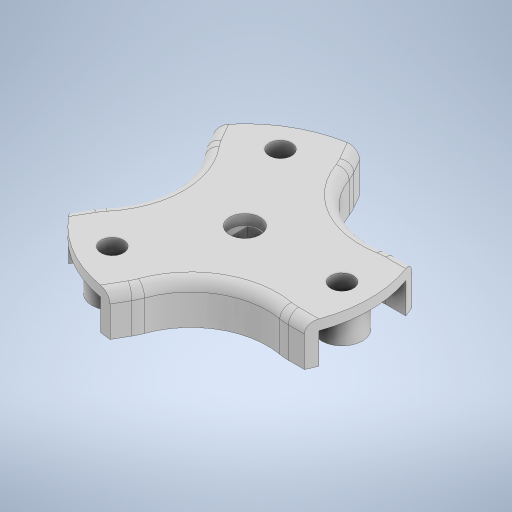
# Autodesk Inventor part: Soporte rodamientos
Saved by Autodesk Inventor 2023 (Build 270158000, 158)
## iProperties
Created: 2023-04-01
Part Number: Soporte rodamientos
Material: Genérico
Document SubType Name: Modeling
Designer: sergi
Density: 1 g/cm^3
Appearance: Valor por defecto
Author: sergi
Autodesk Inventor part; units mm, degrees
ref_plane "YZ Plane" through (0, 0, 0) normal (1, 0, 0) x (0, 1, 0)
ref_plane "XZ Plane" through (0, 0, 0) normal (0, 1, 0) x (-1, 0, 0)
ref_plane "XY Plane" through (0, 0, 0) normal (0, 0, 1) x (1, 0, 0)
sketch "Boceto1" plane through (0, 0, 0) normal (0, 1, 0) x (-1, 0, 0)
  circle A0 centre (0, 0) radius 24.5
  dimension "d0" = 49
  constraints: 1 centre point, 1 coincident
  measures "d0" diameter of A0
extrude "Extrusión1" add sketch "Boceto1" along normal blind 8
sketch "Boceto2" plane through (0, 8, 0) normal (0, 1, 0) x (1, 0, 0)
  circle A0 centre (0, 0) radius 2.65
  line L0 (0, 0) -> (-1.6, 0)
  line L1 (-1.6, 0) -> (-1.6, -2.1125)
  line L2 (-1.6, 2.1125) -> (-1.6, 0)
  line L3 (1.4133, 2.2416) -> (1.4133, -2.2416)
  dimension "d3" = 5.3
  dimension "d4" = 1.6
  constraints: 8 end point, 4 point on circle, 1 centre point, 1 coincident, 1 collinear, 1 horizontal, 1 parallel, 1 perpendicular, 1 point on line
  measures "d3" diameter of A0
  measures "d4" distance of L0.start L0.end
extrude "Extrusión2" cut sketch "Boceto2" against normal through all contours L3 A0 L1 L2
sketch "Boceto3" plane through (0, 8, 0) normal (0, 1, 0) x (1, 0, 0)
  circle A0 centre (0, 0) radius 3
  constraints: 1 centre point, 1 coincident
extrude "Extrusión3" cut sketch "Boceto3" against normal blind 2
sketch "Boceto5" plane through (0, 0, 0) normal (0, -1, 0) x (1, 0, 0)
  line L0 (0, 0) -> (27, 0)
  line L1 (27, 0) -> (19, 0)
  circle A0 centre (19, 0) radius 8.5
  circle A1 centre (19, 0) radius 4
  line L2 (19, -8.5) -> (27.5, -8.5)
  line L3 (27.5, -8.5) -> (27.5, 8.5)
  line L4 (27.5, 8.5) -> (19, 8.5)
  point P0 (27.5, 0)
  dimension "d12" = 27
  dimension "d13" = 8
  dimension "d14" = 17
  dimension "d15" = 8
  constraints: 10 end point, 2 centre point, 2 coincident, 2 horizontal, 2 perpendicular, 2 point on circle, 1 point on line, 1 tangent
  measures "d12" distance of L0.start L0.end
  measures "d13" distance of L0.end L1.end
  measures "d14" diameter of A0
  measures "d15" diameter of A1
extrude "Extrusión4" cut sketch "Boceto5" against normal blind 6
pattern_circular "Patrón circular1" count 3 over 360 about axis through (0, 0, 0) along (0, 1, 0) of "Extrusión4"
sketch "Boceto7" plane through (-9.5, 0, -16.4545) normal (0, -1, 0) x (1, 0, 0)
  circle A0 centre (0, 0) radius 4 projected
  circle A1 centre (0, 32.909) radius 4 projected
  circle A2 centre (28.5, 16.4545) radius 4 projected
  point P0 (9.5, 16.4545)
  constraints: 3 coincident
hole "Agujero1" at (-9.5, 0, -16.4545) at (-9.5, 0, 16.4545) at (19, 0, 0) direction (0, 1, 0) diameter 4.4 end through all
sketch "Boceto8" plane through (0, 0, 0) normal (0, -1, 0) x (1, 0, 0)
  line L0 (-1.6, -2.1125) -> (-1.6, 2.1125) projected
  arc A0 (1.4133, 2.2416) -> (-1.6, 2.1125) centre (0, 0) ccw projected
  line L1 (1.4133, 2.2416) -> (1.4133, -2.2416) projected
  arc A1 (-1.6, -2.1125) -> (1.4133, -2.2416) centre (0, 0) ccw projected
  line L2 (-4.1279, 24.1497) -> (-2.1388, 20.7045) projected
  arc A2 (-16.8612, 12.2045) -> (-2.1388, 20.7045) centre (-9.5, 16.4545) ccw projected
  line L3 (-16.8612, 12.2045) -> (-18.8503, 15.6497) projected
  arc A3 (-18.8503, 15.6497) -> (-18.8503, -15.6497) centre (0, 0) ccw projected
  line L4 (-18.8503, -15.6497) -> (-16.8612, -12.2045) projected
  arc A4 (-2.1388, -20.7045) -> (-16.8612, -12.2045) centre (-9.5, -16.4545) ccw projected
  line L5 (-2.1388, -20.7045) -> (-4.1279, -24.1497) projected
  arc A5 (-4.1279, -24.1497) -> (22.9783, -8.5) centre (0, 0) ccw projected
  line L6 (22.9783, -8.5) -> (19, -8.5) projected
  arc A6 (19, 8.5) -> (19, -8.5) centre (19, 0) ccw projected
  line L7 (19, 8.5) -> (22.9783, 8.5) projected
  arc A7 (22.9783, 8.5) -> (-4.1279, 24.1497) centre (0, 0) ccw projected
  arc A8 (-0.8566, -22.4837) -> (19.8997, -10.5) centre (0, 0) ccw
  line L8 (-1.9747, -24.4203) -> (-0.4067, -21.7045)
  arc A9 (-0.4067, -21.7045) -> (-18.5933, -11.2045) centre (-9.5, -16.4545) ccw
  line L9 (-18.5933, -11.2045) -> (-20.1612, -13.9203)
  arc A10 (-19.0431, 11.9837) -> (-19.0431, -11.9837) centre (0, 0) ccw
  line L10 (-20.1612, 13.9203) -> (-18.5933, 11.2045)
  arc A11 (-18.5933, 11.2045) -> (-0.4067, 21.7045) centre (-9.5, 16.4545) ccw
  line L11 (-0.4067, 21.7045) -> (-1.9747, 24.4203)
  arc A12 (19.8997, 10.5) -> (-0.8566, 22.4837) centre (0, 0) ccw
  line L12 (22.1359, 10.5) -> (19, 10.5)
  arc A13 (19, 10.5) -> (19, -10.5) centre (19, 0) ccw
  line L13 (19, -10.5) -> (22.1359, -10.5)
  circle A14 centre (-28.9808, 0) radius 15
  circle A15 centre (14.4904, -25.0981) radius 15
  circle A16 centre (14.4904, 25.0981) radius 15
  point P0 (17.1431, -10.3345)
  point P1 (0.3784, -20.0136)
  point P2 (-20.9645, 12.6783)
  point P3 (-20.9645, -12.6783)
  point P4 (-17.5215, -9.6791)
  point P5 (-17.5215, 9.6791)
  point P6 (17.1431, 10.3345)
  point P7 (0.3784, 20.0136)
  dimension "d28" = 2
  dimension "d29" = 30
  dimension "d30" = 30
  dimension "d31" = 30
  constraints: 18 point on circle, 12 end point, 9 centre point, 6 point on line, 6 tangent
  measures "d28" radial gap between concentric circles of A5 A8
  measures "d29" diameter of A14
  measures "d30" diameter of A15
  measures "d31" diameter of A16
extrude "Extrusión5" cut sketch "Boceto8" against normal through all contours A7 A16 A12 L11 | A7 A16 A12 | A12 A16 A11 L11 | A7 L12 A12 A16 | A12 A16 | L10 A10 A14 A3 | A12 L12 A13 A16 | A14 A10 A3 | A3 A14 | L10 A11 A14 A10 | A14 A10 | A14 A10 L9 A3 | A13 L13 A8 A15 | A15 A8 | A14 A9 L9 A10 | A15 A5 A8 | A8 L13 A5 A15 | A15 A8 L8 A9 | A15 A5 L8 A8
fillet "Empalme1" radius 2 15 edges at (18.0679, 8, 10.4585) (6.9904, 8, 12.1077) (0.0234, 8, 20.8765) (-1.1907, 8, 23.0624) (20.568, 8, 10.5) (-18.0913, 8, 10.418) (-19.3773, 8, 12.5624) (-18.0913, 8, -10.418) (-19.3773, 8, -12.5624) (-13.9808, 8, 0) (0.0234, 8, -20.8765) (-1.1907, 8, -23.0624) (18.0679, 8, -10.4585) (20.568, 8, -10.5) (6.9904, 8, -12.1077)
